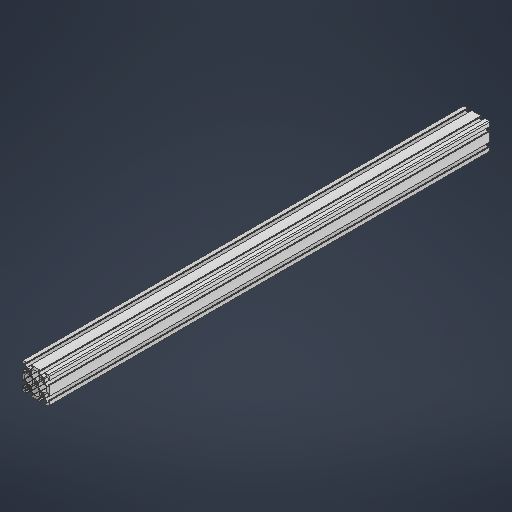
# Autodesk Inventor part: 20-2020-285
Saved by Autodesk Inventor 2026.2 (Build 302298000, 298)
## iProperties
Created: 2024-06-13
Part Number: 20-2020-285
Material: Generic
Document SubType Name: Modeling
Designer: mumin
Density: 1 g/cm^3
Appearance: Default
Author: mumin
Autodesk Inventor part; units mm, degrees
ref_plane "YZ Plane" through (0, 0, 0) normal (1, 0, 0) x (0, 1, 0)
ref_plane "XZ Plane" through (0, 0, 0) normal (0, 1, 0) x (-1, 0, 0)
ref_plane "XY Plane" through (0, 0, 0) normal (0, 0, 1) x (1, 0, 0)
sketch "Sketch1" plane through (0, 0, 0) normal (0, 0, 1) x (1, 0, 0)
  arc A0 (-20.0002, -18.5026) -> (-18.5002, -20.0026) centre (-18.5002, -18.5026) ccw
  line L0 (-18.5002, -20.0026) -> (-13.1382, -20.0026)
  arc A1 (-13.1382, -20.0026) -> (-12.6302, -19.4946) centre (-13.1382, -19.4946) ccw
  line L1 (-12.6302, -19.4946) -> (-12.6302, -19.0106)
  arc A2 (-12.6302, -19.0106) -> (-13.1382, -18.5026) centre (-13.1382, -19.0106) ccw
  line L2 (-13.1382, -18.5026) -> (-15.4872, -18.5026)
  arc A3 (-15.9952, -17.9946) -> (-15.4872, -18.5026) centre (-15.4872, -17.9946) ccw
  line L3 (-15.9952, -17.9946) -> (-15.9952, -17.2689)
  arc A4 (-15.8464, -16.9097) -> (-15.9952, -17.2689) centre (-15.4872, -17.2689) ccw
  line L4 (-15.8464, -16.9097) -> (-12.7431, -13.8064)
  arc A5 (-12.3839, -13.6576) -> (-12.7431, -13.8064) centre (-12.3839, -14.1656) ccw
  line L5 (-12.3839, -13.6576) -> (-7.6161, -13.6576)
  arc A6 (-7.2569, -13.8064) -> (-7.6161, -13.6576) centre (-7.6161, -14.1656) ccw
  line L6 (-7.2569, -13.8064) -> (-4.1539, -16.9093)
  arc A7 (-4.0052, -17.2685) -> (-4.1539, -16.9093) centre (-4.5132, -17.2685) ccw
  line L7 (-4.0052, -17.2685) -> (-4.0052, -17.9946)
  arc A8 (-4.5132, -18.5026) -> (-4.0052, -17.9946) centre (-4.5132, -17.9946) ccw
  line L8 (-4.5132, -18.5026) -> (-6.8622, -18.5026)
  arc A9 (-6.8622, -18.5026) -> (-7.3702, -19.0106) centre (-6.8622, -19.0106) ccw
  line L9 (-7.3702, -19.0106) -> (-7.3702, -19.4946)
  arc A10 (-7.3702, -19.4946) -> (-6.8622, -20.0026) centre (-6.8622, -19.4946) ccw
  line L10 (-6.8622, -20.0026) -> (-1.5002, -20.0026)
  line L11 (-2.0081, -15.9977) -> (-2.7338, -15.9977)
  arc A11 (-3.093, -15.8489) -> (-2.7338, -15.9977) centre (-2.7338, -15.4897) ccw
  line L12 (-3.093, -15.8489) -> (-6.1963, -12.7456)
  arc A12 (-6.3451, -12.3864) -> (-6.1963, -12.7456) centre (-5.8371, -12.3864) ccw
  line L13 (-6.3451, -12.3864) -> (-6.3451, -7.6186)
  arc A13 (-6.1963, -7.2594) -> (-6.3451, -7.6186) centre (-5.8371, -7.6186) ccw
  line L14 (-6.1963, -7.2594) -> (-3.0933, -4.1564)
  arc A14 (-2.7341, -4.0077) -> (-3.0933, -4.1564) centre (-2.7341, -4.5157) ccw
  line L15 (-2.7341, -4.0077) -> (-2.0081, -4.0077)
  line L16 (-4.005, 2.001) -> (-4.0051, -2.7364)
  arc A15 (-4.1539, -3.0956) -> (-4.0051, -2.7364) centre (-4.5131, -2.7364) ccw
  line L17 (-4.1539, -3.0956) -> (-7.2571, -6.1988)
  arc A16 (-7.6163, -6.3477) -> (-7.2571, -6.1988) centre (-7.6163, -5.8397) ccw
  line L18 (-7.6163, -6.3477) -> (-12.3841, -6.3477)
  arc A17 (-12.7433, -6.1989) -> (-12.3841, -6.3477) centre (-12.3841, -5.8397) ccw
  line L19 (-12.7433, -6.1989) -> (-15.8463, -3.0959)
  arc A18 (-15.9951, -2.7367) -> (-15.8463, -3.0959) centre (-15.4871, -2.7367) ccw
  line L20 (-15.9951, -2.7367) -> (-15.9951, -2.0107)
  arc A19 (-15.995, -2.0054) -> (-15.9951, -2.0107) centre (-15.4871, -2.0107) ccw
  line L21 (-20.0002, 6.8646) -> (-20.0002, -6.8646)
  arc A20 (-20.0002, -6.8646) -> (-19.4922, -7.3726) centre (-19.4922, -6.8646) ccw
  line L22 (-19.4922, -7.3726) -> (-19.0082, -7.3726)
  arc A21 (-19.0082, -7.3726) -> (-18.5002, -6.8646) centre (-19.0082, -6.8646) ccw
  line L23 (-18.5002, -6.8646) -> (-18.5002, -4.5156)
  arc A22 (-17.9922, -4.0076) -> (-18.5002, -4.5156) centre (-17.9922, -4.5156) ccw
  line L24 (-17.9922, -4.0076) -> (-17.2664, -4.0076)
  arc A23 (-16.9072, -4.1564) -> (-17.2664, -4.0076) centre (-17.2664, -4.5156) ccw
  line L25 (-16.9072, -4.1564) -> (-13.8039, -7.2597)
  arc A24 (-13.6552, -7.6189) -> (-13.8039, -7.2597) centre (-14.1632, -7.6189) ccw
  line L26 (-13.6552, -7.6189) -> (-13.6552, -12.3867)
  arc A25 (-13.8039, -12.7459) -> (-13.6552, -12.3867) centre (-14.1632, -12.3867) ccw
  line L27 (-13.8039, -12.7459) -> (-16.9069, -15.8488)
  arc A26 (-17.2661, -15.9976) -> (-16.9069, -15.8488) centre (-17.2661, -15.4896) ccw
  line L28 (-17.2661, -15.9976) -> (-17.9922, -15.9976)
  arc A27 (-18.5002, -15.4896) -> (-17.9922, -15.9976) centre (-17.9922, -15.4896) ccw
  line L29 (-18.5002, -15.4896) -> (-18.5002, -13.1406)
  arc A28 (-18.5002, -13.1406) -> (-19.0082, -12.6326) centre (-19.0082, -13.1406) ccw
  line L30 (-19.0082, -12.6326) -> (-19.4922, -12.6326)
  arc A29 (-19.4922, -12.6326) -> (-20.0002, -13.1406) centre (-19.4922, -13.1406) ccw
  line L31 (-20.0002, -13.1406) -> (-20.0002, -18.5026)
  arc A30 (-11.9359, -10.8064) -> (-12.3047, -12.1271) centre (-11.7482, -11.5706) ccw
  line L32 (-12.3047, -12.1271) -> (-12.1247, -12.3071)
  arc A31 (-12.1247, -12.3071) -> (-10.8039, -11.9384) centre (-11.5682, -11.7506) ccw
  arc A32 (-10.8039, -11.9384) -> (-9.1964, -11.9384) centre (-10.0002, -10.0026) ccw
  arc A33 (-9.1964, -11.9384) -> (-7.8757, -12.3071) centre (-8.4322, -11.7506) ccw
  line L33 (-7.8757, -12.3071) -> (-7.6957, -12.1271)
  arc A34 (-7.6957, -12.1271) -> (-8.0644, -10.8064) centre (-8.2522, -11.5706) ccw
  arc A35 (-8.0644, -10.8064) -> (-8.0644, -9.1989) centre (-10.0002, -10.0026) ccw
  arc A36 (-8.0644, -9.1989) -> (-7.6957, -7.8781) centre (-8.2522, -8.4346) ccw
  line L34 (-7.6957, -7.8781) -> (-7.8757, -7.6981)
  arc A37 (-7.8757, -7.6981) -> (-9.1964, -8.0668) centre (-8.4322, -8.2546) ccw
  arc A38 (-9.1964, -8.0668) -> (-10.8039, -8.0668) centre (-10.0002, -10.0026) ccw
  arc A39 (-10.8039, -8.0668) -> (-12.1247, -7.6981) centre (-11.5682, -8.2546) ccw
  line L35 (-12.1247, -7.6981) -> (-12.3047, -7.8781)
  arc A40 (-12.3047, -7.8781) -> (-11.9359, -9.1989) centre (-11.7482, -8.4346) ccw
  arc A41 (-11.9359, -9.1989) -> (-11.9359, -10.8064) centre (-10.0002, -10.0026) ccw
  arc A42 (-18.5002, 4.5104) -> (-17.9922, 4.0024) centre (-17.9922, 4.5104) ccw
  line L36 (-17.2661, 4.0024) -> (-17.9922, 4.0024)
  arc A43 (-17.2661, 4.0024) -> (-16.9068, 4.1511) centre (-17.2659, 4.5104) ccw
  line L37 (-15.995, -2.0054) -> (-15.995, 2.7311)
  arc A44 (-15.8464, 3.0903) -> (-15.995, 2.7311) centre (-15.487, 2.7313) ccw
  line L38 (-13.8038, 7.2541) -> (-16.9068, 4.1511)
  line L39 (-15.8464, 3.0903) -> (-12.7431, 6.1936)
  arc A45 (-18.5002, 6.8594) -> (-19.0082, 7.3674) centre (-19.0082, 6.8594) ccw
  arc A46 (-19.4922, 7.3674) -> (-20.0002, 6.8594) centre (-19.4922, 6.8594) ccw
  line L40 (-19.0082, 7.3674) -> (-19.4922, 7.3674)
  line L41 (-18.5002, 4.5104) -> (-18.5002, 6.8594)
  arc A47 (-7.2569, 6.1936) -> (-7.6161, 6.3424) centre (-7.6161, 5.8344) ccw
  line L42 (-7.2569, 6.1936) -> (-4.154, 3.0907)
  arc A48 (-4.005, 2.7304) -> (-4.154, 3.0907) centre (-4.513, 2.7313) ccw
  line L43 (-4.005, 2.7304) -> (-4.005, 2.0043)
  line L44 (-2.0081, 4.0023) -> (-2.7338, 4.0023)
  arc A49 (-3.093, 4.1511) -> (-2.7338, 4.0023) centre (-2.7338, 4.5103) ccw
  line L45 (-3.093, 4.1511) -> (-6.1963, 7.2544)
  arc A50 (-4.0051, 2.0001) -> (-4.005, 2.0043) centre (-4.513, 2.0043) ccw
  arc A51 (-12.3839, 6.3424) -> (-12.7431, 6.1936) centre (-12.3839, 5.8344) ccw
  line L46 (-12.3839, 6.3424) -> (-7.6161, 6.3424)
  line L47 (-7.8757, 7.692) -> (-7.6957, 7.872)
  arc A52 (-7.6957, 7.872) -> (-8.0644, 9.1927) centre (-8.2522, 8.4285) ccw
  arc A53 (-9.1964, 8.0607) -> (-7.8757, 7.692) centre (-8.4322, 8.2485) ccw
  arc A54 (-10.8039, 8.0607) -> (-9.1964, 8.0607) centre (-10.0002, 9.9965) ccw
  line L48 (-12.3047, 7.872) -> (-12.1247, 7.692)
  arc A55 (-11.9359, 9.1927) -> (-12.3047, 7.872) centre (-11.7482, 8.4285) ccw
  arc A56 (-12.1247, 7.692) -> (-10.8039, 8.0607) centre (-11.5682, 8.2485) ccw
  arc A57 (-7.3702, 19.0054) -> (-6.8622, 18.4974) centre (-6.8622, 19.0054) ccw
  arc A58 (-6.8622, 19.9974) -> (-7.3702, 19.4894) centre (-6.8622, 19.4894) ccw
  line L49 (-7.3702, 19.4894) -> (-7.3702, 19.0054)
  arc A59 (-6.1964, 12.7407) -> (-6.3451, 12.3814) centre (-5.8371, 12.3816) ccw
  arc A60 (-7.6163, 13.6523) -> (-7.2571, 13.8011) centre (-7.6163, 14.1603) ccw
  line L50 (-6.1964, 12.7407) -> (-3.0935, 15.8436)
  arc A61 (-2.7342, 15.9924) -> (-3.0935, 15.8436) centre (-2.7342, 15.4844) ccw
  line L51 (-6.8622, 18.4974) -> (-4.5132, 18.4974)
  arc A62 (-4.0051, 17.9893) -> (-4.5132, 18.4974) centre (-4.5131, 17.9894) ccw
  line L52 (-4.0051, 17.9893) -> (-4.0051, 17.2636)
  arc A63 (-4.1538, 16.9044) -> (-4.0051, 17.2636) centre (-4.5131, 17.2636) ccw
  line L53 (-1.5002, 19.9974) -> (-6.8622, 19.9974)
  line L54 (-2.7342, 15.9924) -> (-2.0082, 15.9924)
  line L55 (-4.1538, 16.9044) -> (-7.2571, 13.8011)
  arc A64 (-6.3451, 7.6136) -> (-6.1963, 7.2544) centre (-5.8371, 7.6136) ccw
  line L56 (-6.3451, 7.6136) -> (-6.3451, 12.3814)
  line L57 (-7.6957, 12.1209) -> (-7.8757, 12.3009)
  arc A65 (-7.8757, 12.3009) -> (-9.1964, 11.9322) centre (-8.4322, 11.7445) ccw
  arc A66 (-8.0644, 10.8002) -> (-7.6957, 12.1209) centre (-8.2522, 11.5645) ccw
  arc A67 (-9.1964, 11.9322) -> (-10.8039, 11.9322) centre (-10.0002, 9.9965) ccw
  arc A68 (-8.0644, 9.1927) -> (-8.0644, 10.8002) centre (-10.0002, 9.9965) ccw
  line L58 (-7.6163, 13.6523) -> (-12.3841, 13.6523)
  line L59 (-12.7433, 13.8011) -> (-15.8463, 16.9041)
  arc A69 (-15.9951, 17.2633) -> (-15.8463, 16.9041) centre (-15.4871, 17.2633) ccw
  line L60 (-15.9951, 17.2633) -> (-15.9951, 17.9893)
  arc A70 (-16.9071, 15.8436) -> (-17.2663, 15.9923) centre (-17.2663, 15.4843) ccw
  arc A71 (-17.9921, 15.9923) -> (-18.5001, 15.4843) centre (-17.9921, 15.4843) ccw
  line L61 (-16.9071, 15.8436) -> (-13.8038, 12.7403)
  line L62 (-20.0001, 18.4973) -> (-20.0001, 13.1353)
  line L63 (-18.5001, 13.1353) -> (-18.5001, 15.4843)
  arc A72 (-19.0081, 12.6273) -> (-18.5001, 13.1353) centre (-19.0081, 13.1353) ccw
  line L64 (-19.4921, 12.6273) -> (-19.0081, 12.6273)
  arc A73 (-20.0001, 13.1353) -> (-19.4921, 12.6273) centre (-19.4921, 13.1353) ccw
  line L65 (-17.9921, 15.9923) -> (-17.2663, 15.9923)
  arc A74 (-15.4871, 18.4973) -> (-15.9951, 17.9893) centre (-15.4871, 17.9893) ccw
  arc A75 (-18.5001, 19.9973) -> (-20.0001, 18.4973) centre (-18.5001, 18.4973) ccw
  line L66 (-13.1381, 19.9973) -> (-18.5001, 19.9973)
  line L67 (-15.4871, 18.4973) -> (-13.1381, 18.4973)
  arc A76 (-12.7433, 13.8011) -> (-12.3841, 13.6523) centre (-12.3841, 14.1603) ccw
  arc A77 (-13.6551, 12.3811) -> (-13.8038, 12.7403) centre (-14.1631, 12.3811) ccw
  arc A78 (-13.1381, 18.4973) -> (-12.6301, 19.0053) centre (-13.1381, 19.0053) ccw
  line L68 (-12.6301, 19.0053) -> (-12.6301, 19.4893)
  arc A79 (-12.6301, 19.4893) -> (-13.1381, 19.9973) centre (-13.1381, 19.4893) ccw
  arc A80 (-13.8038, 7.2541) -> (-13.6551, 7.6133) centre (-14.1631, 7.6133) ccw
  line L69 (-12.1247, 12.3009) -> (-12.3047, 12.1209)
  arc A81 (-12.3047, 12.1209) -> (-11.9359, 10.8002) centre (-11.7482, 11.5645) ccw
  arc A82 (-10.8039, 11.9322) -> (-12.1247, 12.3009) centre (-11.5682, 11.7445) ccw
  line L70 (-13.6551, 12.3811) -> (-13.6551, 7.6133)
  arc A83 (-11.9359, 10.8002) -> (-11.9359, 9.1927) centre (-10.0002, 9.9965) ccw
  arc A84 (-18.8882, -0.0537) -> (-18.8884, -0.0538) centre (-18.5002, -1.5026) ccw
  arc A85 (-19.0398, -0.103) -> (-19.0403, -0.1032) centre (-18.5002, -1.5026) ccw
  arc A86 (-19.949, 1.1092) -> (-19.9489, 1.109) centre (-18.5001, 1.4973) ccw
  arc A87 (-19.8996, 0.9577) -> (-19.8994, 0.9572) centre (-18.5001, 1.4973) ccw
  arc A88 (-19.8996, -0.9625) -> (-19.8998, -0.963) centre (-18.5002, -1.5026) ccw
  arc A89 (-19.949, -1.1143) -> (-19.9491, -1.1145) centre (-18.5002, -1.5026) ccw
  arc A90 (-19.0402, 0.098) -> (-19.0397, 0.0978) centre (-18.5001, 1.4973) ccw
  arc A91 (-18.8885, 0.0485) -> (-18.8883, 0.0485) centre (-18.5001, 1.4973) ccw
  line L71 (-18.4937, -0.0027) -> (-18.5002, -0.0027)
  line L72 (-18.5002, -0.0027) -> (-18.4937, -0.0027)
  arc A92 (17.9922, -15.9976) -> (18.5002, -15.4896) centre (17.9922, -15.4896) ccw
  line L73 (17.2661, -15.9976) -> (17.9922, -15.9976)
  arc A93 (16.9069, -15.8488) -> (17.2661, -15.9976) centre (17.2661, -15.4896) ccw
  line L74 (15.9952, -17.9946) -> (15.9952, -17.2689)
  arc A94 (15.9952, -17.2689) -> (15.8464, -16.9097) centre (15.4872, -17.2689) ccw
  arc A95 (15.4872, -18.5026) -> (15.9952, -17.9946) centre (15.4872, -17.9946) ccw
  line L75 (13.804, -12.7459) -> (16.9069, -15.8488)
  line L76 (18.5002, -20.0026) -> (13.1382, -20.0026)
  line L77 (13.1382, -18.5026) -> (15.4872, -18.5026)
  arc A96 (13.1382, -18.5026) -> (12.6302, -19.0106) centre (13.1382, -19.0106) ccw
  line L78 (12.6302, -19.4946) -> (12.6302, -19.0106)
  arc A97 (12.6302, -19.4946) -> (13.1382, -20.0026) centre (13.1382, -19.4946) ccw
  line L79 (15.8464, -16.9097) -> (12.7431, -13.8064)
  arc A98 (19.0082, -12.6326) -> (18.5002, -13.1406) centre (19.0082, -13.1406) ccw
  arc A99 (20.0002, -13.1406) -> (19.4922, -12.6326) centre (19.4922, -13.1406) ccw
  line L80 (19.0082, -12.6326) -> (19.4922, -12.6326)
  arc A100 (18.5002, -20.0026) -> (20.0002, -18.5026) centre (18.5002, -18.5026) ccw
  line L81 (18.5002, -15.4896) -> (18.5002, -13.1406)
  line L82 (20.0002, -13.1406) -> (20.0002, -18.5026)
  arc A101 (7.6161, -13.6576) -> (7.2569, -13.8064) centre (7.6161, -14.1656) ccw
  line L83 (7.2569, -13.8064) -> (4.154, -16.9093)
  arc A102 (4.154, -16.9093) -> (4.0052, -17.2685) centre (4.5132, -17.2685) ccw
  line L84 (4.0052, -17.2685) -> (4.0052, -17.9946)
  line L85 (2.0083, -15.9977) -> (2.7341, -15.9977)
  arc A103 (2.7341, -15.9977) -> (3.0932, -15.8488) centre (2.7339, -15.4897) ccw
  line L86 (3.0932, -15.8488) -> (6.1964, -12.7456)
  arc A104 (4.0052, -17.9946) -> (4.5132, -18.5026) centre (4.5132, -17.9946) ccw
  line L87 (4.5132, -18.5026) -> (6.8622, -18.5026)
  line L88 (6.8622, -20.0026) -> (1.5002, -20.0026)
  arc A105 (12.7431, -13.8064) -> (12.3839, -13.6576) centre (12.3839, -14.1656) ccw
  line L89 (12.3839, -13.6576) -> (7.6161, -13.6576)
  line L90 (7.8757, -12.3071) -> (7.6957, -12.1271)
  arc A106 (8.0644, -10.8064) -> (7.6957, -12.1271) centre (8.2522, -11.5706) ccw
  arc A107 (7.8757, -12.3071) -> (9.1964, -11.9384) centre (8.4322, -11.7506) ccw
  arc A108 (9.1964, -11.9384) -> (10.8039, -11.9384) centre (10.0002, -10.0026) ccw
  line L91 (12.3047, -12.1271) -> (12.1247, -12.3071)
  arc A109 (12.3047, -12.1271) -> (11.9359, -10.8064) centre (11.7482, -11.5706) ccw
  arc A110 (10.8039, -11.9384) -> (12.1247, -12.3071) centre (11.5682, -11.7506) ccw
  arc A111 (6.3452, -7.6185) -> (6.1965, -7.2594) centre (5.8372, -7.6184) ccw
  arc A112 (7.2572, -6.1988) -> (7.6164, -6.3476) centre (7.6165, -5.8396) ccw
  line L92 (6.1965, -7.2594) -> (3.0936, -4.1564)
  arc A113 (3.0936, -4.1564) -> (2.7344, -4.0077) centre (2.7344, -4.5157) ccw
  line L93 (4.0052, 2.001) -> (4.0052, -2.7364)
  arc A114 (4.0052, -2.7364) -> (4.154, -3.0956) centre (4.5132, -2.7364) ccw
  line L94 (2.7344, -4.0077) -> (2.0083, -4.0077)
  line L95 (4.154, -3.0956) -> (7.2572, -6.1988)
  arc A115 (6.1964, -12.7456) -> (6.3452, -12.3864) centre (5.8372, -12.3864) ccw
  line L96 (6.3452, -12.3864) -> (6.3452, -7.6185)
  line L97 (7.6957, -7.8781) -> (7.8757, -7.6981)
  arc A116 (9.1964, -8.0668) -> (7.8757, -7.6981) centre (8.4322, -8.2546) ccw
  arc A117 (7.6957, -7.8781) -> (8.0644, -9.1989) centre (8.2522, -8.4346) ccw
  arc A118 (10.8039, -8.0668) -> (9.1964, -8.0668) centre (10.0002, -10.0026) ccw
  arc A119 (8.0644, -9.1989) -> (8.0644, -10.8064) centre (10.0002, -10.0026) ccw
  line L98 (7.6164, -6.3476) -> (12.3843, -6.3476)
  line L99 (12.7435, -6.1988) -> (15.8464, -3.0959)
  arc A120 (15.8464, -3.0959) -> (15.9952, -2.7367) centre (15.4872, -2.7367) ccw
  line L100 (15.9952, -2.7367) -> (15.9952, -2.0106)
  arc A121 (17.2664, -4.0076) -> (16.9072, -4.1564) centre (17.2664, -4.5156) ccw
  arc A122 (18.5002, -4.5156) -> (17.9922, -4.0076) centre (17.9922, -4.5156) ccw
  line L101 (16.9072, -4.1564) -> (13.804, -7.2597)
  line L102 (20.0002, 6.8646) -> (20.0002, -6.8646)
  line L103 (18.5002, -6.8646) -> (18.5002, -4.5156)
  arc A123 (18.5002, -6.8646) -> (19.0082, -7.3726) centre (19.0082, -6.8646) ccw
  line L104 (19.4922, -7.3726) -> (19.0082, -7.3726)
  arc A124 (19.4922, -7.3726) -> (20.0002, -6.8646) centre (19.4922, -6.8646) ccw
  line L105 (17.9922, -4.0076) -> (17.2664, -4.0076)
  arc A125 (15.9952, -2.0106) -> (15.9952, -2.0054) centre (15.4872, -2.0095) ccw
  arc A126 (12.3843, -6.3476) -> (12.7435, -6.1988) centre (12.3843, -5.8396) ccw
  arc A127 (13.804, -7.2597) -> (13.6552, -7.6189) centre (14.1632, -7.6189) ccw
  arc A128 (13.6552, -12.3867) -> (13.804, -12.7459) centre (14.1632, -12.3867) ccw
  arc A129 (7.3702, -19.0106) -> (6.8622, -18.5026) centre (6.8622, -19.0106) ccw
  line L106 (7.3702, -19.0106) -> (7.3702, -19.4946)
  arc A130 (6.8622, -20.0026) -> (7.3702, -19.4946) centre (6.8622, -19.4946) ccw
  line L107 (12.1247, -7.6981) -> (12.3047, -7.8781)
  arc A131 (11.9359, -9.1989) -> (12.3047, -7.8781) centre (11.7482, -8.4346) ccw
  arc A132 (12.1247, -7.6981) -> (10.8039, -8.0668) centre (11.5682, -8.2546) ccw
  line L108 (13.6552, -7.6189) -> (13.6552, -12.3867)
  arc A133 (11.9359, -10.8064) -> (11.9359, -9.1989) centre (10.0002, -10.0026) ccw
  line L109 (15.8464, 3.0903) -> (12.7431, 6.1936)
  arc A134 (12.7431, 6.1936) -> (12.3839, 6.3424) centre (12.3839, 5.8344) ccw
  arc A135 (9.1964, 8.0607) -> (10.8039, 8.0607) centre (10.0002, 9.9965) ccw
  arc A136 (7.8757, 7.692) -> (9.1964, 8.0607) centre (8.4322, 8.2485) ccw
  line L110 (12.3839, 6.3424) -> (7.6161, 6.3424)
  arc A137 (6.3452, 12.3815) -> (6.1964, 12.7407) centre (5.8372, 12.3814) ccw
  line L111 (6.3452, 7.6136) -> (6.3452, 12.3815)
  arc A138 (7.6957, 12.1209) -> (8.0644, 10.8002) centre (8.2522, 11.5645) ccw
  arc A139 (8.0644, 10.8002) -> (8.0644, 9.1927) centre (10.0002, 9.9965) ccw
  arc A140 (6.1965, 7.2544) -> (6.3452, 7.6136) centre (5.8372, 7.6134) ccw
  arc A141 (8.0644, 9.1927) -> (7.6957, 7.872) centre (8.2522, 8.4285) ccw
  line L112 (7.8757, 7.692) -> (7.6957, 7.872)
  arc A142 (7.6161, 6.3424) -> (7.2569, 6.1936) centre (7.6161, 5.8344) ccw
  line L113 (7.2569, 6.1936) -> (4.154, 3.0907)
  arc A143 (4.0052, 2.0054) -> (4.0052, 2.0001) centre (4.5132, 2.0054) ccw
  arc A144 (4.154, 3.0907) -> (4.0052, 2.7315) centre (4.5132, 2.7315) ccw
  arc A145 (2.7341, 4.0023) -> (3.0933, 4.1511) centre (2.7341, 4.5103) ccw
  line L114 (3.0933, 4.1511) -> (6.1965, 7.2544)
  line L115 (2.0083, 4.0023) -> (2.7341, 4.0023)
  line L116 (4.0052, 2.7315) -> (4.0052, 2.0054)
  arc A146 (17.9922, 4.0024) -> (18.5002, 4.5104) centre (17.9922, 4.5104) ccw
  line L117 (17.2661, 4.0024) -> (17.9922, 4.0024)
  arc A147 (16.9069, 4.1512) -> (17.2661, 4.0024) centre (17.2661, 4.5104) ccw
  line L118 (15.9952, -2.0054) -> (15.9952, 2.7311)
  arc A148 (15.9952, 2.7311) -> (15.8464, 3.0903) centre (15.4872, 2.7311) ccw
  line L119 (13.804, 7.2541) -> (16.9069, 4.1512)
  line L120 (18.5002, 4.5104) -> (18.5002, 6.8594)
  arc A149 (19.0082, 7.3674) -> (18.5002, 6.8594) centre (19.0082, 6.8594) ccw
  line L121 (19.0082, 7.3674) -> (19.4922, 7.3674)
  arc A150 (20.0002, 6.8594) -> (19.4922, 7.3674) centre (19.4922, 6.8594) ccw
  arc A151 (6.8622, 18.4974) -> (7.3702, 19.0054) centre (6.8622, 19.0054) ccw
  arc A152 (7.3702, 19.4894) -> (6.8622, 19.9974) centre (6.8622, 19.4894) ccw
  line L122 (7.3702, 19.4894) -> (7.3702, 19.0054)
  arc A153 (7.2572, 13.8012) -> (7.6164, 13.6524) centre (7.6164, 14.1604) ccw
  line L123 (7.6957, 12.1209) -> (7.8757, 12.3009)
  arc A154 (9.1964, 11.9322) -> (7.8757, 12.3009) centre (8.4322, 11.7445) ccw
  arc A155 (10.8039, 11.9322) -> (9.1964, 11.9322) centre (10.0002, 9.9965) ccw
  line L124 (7.6164, 13.6524) -> (12.3843, 13.6524)
  arc A156 (13.804, 12.7403) -> (13.6552, 12.3811) centre (14.1632, 12.3811) ccw
  arc A157 (12.3843, 13.6524) -> (12.7435, 13.8012) centre (12.3843, 14.1604) ccw
  line L125 (12.7435, 13.8012) -> (15.8464, 16.9041)
  arc A158 (15.8464, 16.9041) -> (15.9952, 17.2633) centre (15.4872, 17.2633) ccw
  line L126 (15.9952, 17.2633) -> (15.9952, 17.9894)
  line L127 (17.9922, 15.9924) -> (17.2664, 15.9924)
  arc A159 (17.2664, 15.9924) -> (16.9072, 15.8436) centre (17.2664, 15.4844) ccw
  line L128 (16.9072, 15.8436) -> (13.804, 12.7403)
  arc A160 (18.5002, 15.4844) -> (17.9922, 15.9924) centre (17.9922, 15.4844) ccw
  line L129 (20.0002, 18.4974) -> (20.0002, 13.1354)
  line L130 (18.5002, 13.1354) -> (18.5002, 15.4844)
  arc A161 (18.5002, 13.1354) -> (19.0082, 12.6274) centre (19.0082, 13.1354) ccw
  line L131 (19.4922, 12.6274) -> (19.0082, 12.6274)
  arc A162 (19.4922, 12.6274) -> (20.0002, 13.1354) centre (19.4922, 13.1354) ccw
  line L132 (6.8622, 18.4974) -> (4.5132, 18.4974)
  arc A163 (4.5132, 18.4974) -> (4.0052, 17.9894) centre (4.5132, 17.9894) ccw
  line L133 (4.0052, 17.9894) -> (4.0052, 17.2636)
  arc A164 (4.0052, 17.2636) -> (4.154, 16.9044) centre (4.5132, 17.2636) ccw
  line L134 (1.5002, 19.9974) -> (6.8622, 19.9974)
  line L135 (4.154, 16.9044) -> (7.2572, 13.8012)
  arc A165 (3.0935, 15.8436) -> (2.7342, 15.9924) centre (2.7342, 15.4844) ccw
  line L136 (6.1964, 12.7407) -> (3.0935, 15.8436)
  line L137 (2.7342, 15.9924) -> (2.0082, 15.9924)
  arc A166 (20.0002, 18.4974) -> (18.5002, 19.9974) centre (18.5002, 18.4974) ccw
  arc A167 (11.9359, 9.1927) -> (11.9359, 10.8002) centre (10.0002, 9.9965) ccw
  arc A168 (10.8039, 8.0607) -> (12.1247, 7.692) centre (11.5682, 8.2485) ccw
  line L138 (12.3047, 7.872) -> (12.1247, 7.692)
  arc A169 (12.3047, 7.872) -> (11.9359, 9.1927) centre (11.7482, 8.4285) ccw
  arc A170 (12.1247, 12.3009) -> (10.8039, 11.9322) centre (11.5682, 11.7445) ccw
  line L139 (12.1247, 12.3009) -> (12.3047, 12.1209)
  arc A171 (11.9359, 10.8002) -> (12.3047, 12.1209) centre (11.7482, 11.5645) ccw
  arc A172 (13.6552, 7.6133) -> (13.804, 7.2541) centre (14.1632, 7.6133) ccw
  line L140 (13.6552, 12.3811) -> (13.6552, 7.6133)
  arc A173 (15.9952, 17.9894) -> (15.4872, 18.4974) centre (15.4872, 17.9894) ccw
  line L141 (13.1382, 19.9974) -> (18.5002, 19.9974)
  line L142 (15.4872, 18.4974) -> (13.1382, 18.4974)
  arc A174 (12.6302, 19.0054) -> (13.1382, 18.4974) centre (13.1382, 19.0054) ccw
  arc A175 (13.1382, 19.9974) -> (12.6302, 19.4894) centre (13.1382, 19.4894) ccw
  line L143 (12.6302, 19.0054) -> (12.6302, 19.4894)
  arc A176 (18.8885, -0.0538) -> (18.8883, -0.0537) centre (18.5002, -1.5026) ccw
  arc A177 (19.0403, -0.1032) -> (19.0398, -0.103) centre (18.5002, -1.5026) ccw
  arc A178 (19.949, 1.109) -> (19.9491, 1.1093) centre (18.5002, 1.4974) ccw
  arc A179 (19.8996, 0.9573) -> (19.8998, 0.9578) centre (18.5002, 1.4974) ccw
  arc A180 (19.8998, -0.963) -> (19.8995, -0.9625) centre (18.5002, -1.5026) ccw
  arc A181 (19.9491, -1.1145) -> (19.949, -1.1143) centre (18.5002, -1.5026) ccw
  arc A182 (19.0398, 0.0978) -> (19.0403, 0.098) centre (18.5002, 1.4974) ccw
  arc A183 (18.8883, 0.0485) -> (18.8885, 0.0485) centre (18.5002, 1.4974) ccw
  line L144 (18.4937, -0.0026) -> (18.5002, -0.0026)
  line L145 (18.5002, -0.0026) -> (18.4937, -0.0026)
  line L146 (-2.0081, -15.9977) -> (2.0083, -15.9977)
  line L147 (2.0083, -4.0077) -> (-2.0081, -4.0077)
  line L148 (-2.0081, 4.0023) -> (2.0083, 4.0023)
  line L149 (-2.0082, 15.9924) -> (2.0082, 15.9924)
  line L150 (-1.5002, -20.0026) -> (1.5002, -20.0026)
  line L151 (-1.5002, 19.9974) -> (1.5002, 19.9974)
  arc A184 (-0.9595, 19.8965) -> (-0.96, 19.8967) centre (-1.5002, 18.4974) ccw
  arc A185 (0.96, 19.8967) -> (0.9595, 19.8965) centre (1.5002, 18.4974) ccw
  arc A186 (1.5002, 19.9974) -> (1.4898, 19.9973) centre (1.5002, 18.4974) ccw
  arc A187 (1.1121, 19.9463) -> (1.1118, 19.9462) centre (1.5002, 18.4974) ccw
  arc A188 (2.1245, 2.3045) -> (0.8037, 1.9358) centre (1.568, 1.748) ccw
  line L152 (2.1245, 2.3045) -> (2.3045, 2.1245)
  arc A189 (1.9358, 0.8037) -> (2.3045, 2.1245) centre (1.748, 1.568) ccw
  line L153 (-2.1245, -2.3045) -> (-2.3045, -2.1245)
  line L154 (2.3045, -2.1245) -> (2.1245, -2.3045)
  arc A190 (1.9358, -0.8037) -> (1.9358, 0.8037) centre (0, 0) ccw
  arc A191 (2.3045, -2.1245) -> (1.9358, -0.8037) centre (1.748, -1.568) ccw
  arc A192 (0.8037, -1.9358) -> (2.1245, -2.3045) centre (1.568, -1.748) ccw
  arc A193 (-0.8037, -1.9358) -> (0.8037, -1.9358) centre (0, 0) ccw
  arc A194 (-2.1245, -2.3045) -> (-0.8037, -1.9358) centre (-1.568, -1.748) ccw
  arc A195 (0.8037, 1.9358) -> (-0.8037, 1.9358) centre (0, 0) ccw
  arc A196 (-0.8037, 1.9358) -> (-2.1245, 2.3045) centre (-1.568, 1.748) ccw
  line L155 (-2.3045, 2.1245) -> (-2.1245, 2.3045)
  arc A197 (-1.9358, 0.8037) -> (-1.9358, -0.8037) centre (0, 0) ccw
  arc A198 (-2.3045, 2.1245) -> (-1.9358, 0.8037) centre (-1.748, 1.568) ccw
  arc A199 (-1.9358, -0.8037) -> (-2.3045, -2.1245) centre (-1.748, -1.568) ccw
  point P0 (0, 0)
  point P1 (0, -15.9977)
  point P2 (-6.3451, -0.0027)
  point P3 (-6.3451, -1.5027)
  point P4 (-20.0002, -1.5026)
  point P5 (-0.0002, 15.9924)
  point P6 (10.0002, -10.0026)
  point P7 (6.3452, -0.0026)
  point P8 (6.3452, -1.5026)
  point P9 (20.0002, -1.5026)
  constraints: 406 point on circle, 312 end point, 200 centre point, 51 point on line, 4 parallel, 2 horizontal, 1 tangent
extrude "Extrusion2" add sketch "Sketch1" along normal mid plane 650
body "Solid2"
